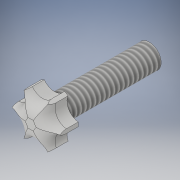
# Autodesk Inventor part: Bike Seat Bolt
Saved by Autodesk Inventor 2019 (Build 230136000, 136)
## iProperties
Created: 2020-05-31
Part Number: Bike Seat Bolt
Material: Generic
Document SubType Name: Modeling
Designer: 18186
Density: 1 g/cm^3
Appearance: Default
Author: 18186
Autodesk Inventor part; units mm, degrees
ref_plane "YZ Plane" through (0, 0, 0) normal (1, 0, 0) x (0, 1, 0)
ref_plane "XZ Plane" through (0, 0, 0) normal (0, 1, 0) x (-1, 0, 0)
ref_plane "XY Plane" through (0, 0, 0) normal (0, 0, 1) x (1, 0, 0)
sketch "Sketch1" plane through (0, 0, 0) normal (0, 0, 1) x (1, 0, 0)
  circle A0 centre (0, 0) radius 3.175
  dimension "d0" = 6.35
  constraints: 1 centre point, 1 coincident
  measures "d0" diameter of A0
extrude "Extrusion1" add sketch "Sketch1" along normal blind 25.4
sketch "Sketch2" plane through (0, 0, 25.4) normal (0, 0, 1) x (1, 0, 0)
  arc A0 (-2.7118, 5.7968) -> (2.7118, 5.7968) centre (0, 7.7132) ccw
  arc A1 (-6.3761, 0.5499) -> (-3.6643, 5.2469) centre (-6.6798, 3.8566) ccw
  arc A2 (-3.6643, -5.2469) -> (-6.3761, -0.5499) centre (-6.6798, -3.8566) ccw
  arc A3 (2.7118, -5.7968) -> (-2.7118, -5.7968) centre (0, -7.7132) ccw
  arc A4 (6.3761, -0.5499) -> (3.6643, -5.2469) centre (6.6798, -3.8566) ccw
  arc A5 (3.6643, 5.2469) -> (6.3761, 0.5499) centre (6.6798, 3.8566) ccw
  arc A6 (-2.7118, 5.7968) -> (-3.6643, 5.2469) centre (0, 0) ccw
  arc A7 (3.6643, 5.2469) -> (2.7118, 5.7968) centre (0, 0) ccw
  arc A8 (6.3761, -0.5499) -> (6.3761, 0.5499) centre (0, 0) ccw
  arc A9 (2.7118, -5.7968) -> (3.6643, -5.2469) centre (0, 0) ccw
  arc A10 (-6.3761, 0.5499) -> (-6.3761, -0.5499) centre (0, 0) ccw
  arc A11 (-3.6643, -5.2469) -> (-2.7118, -5.7968) centre (0, 0) ccw
  point P0 (-6.3761, -0.5499)
  point P1 (-2.7118, -5.7968)
  point P2 (3.6643, -5.2469)
  point P3 (6.3761, 0.5499)
  point P4 (2.7118, 5.7968)
  dimension "d7" = 360
  constraints: 24 point on circle, 12 centre point, 2 coincident, 25 other
extrude "Extrusion2" add sketch "Sketch2" along normal blind 6.35
fillet "Fillet1" radius 3.175 6 edges at (0, 4.3926, 31.75) (-3.8041, 2.1963, 31.75) (-3.8041, -2.1963, 31.75) (0, -4.3926, 31.75) (3.8041, -2.1963, 31.75) (3.8041, 2.1963, 31.75)
thread "Thread1" size "1/4-20 UNC" class "2A" standard "ANSI Unified Screw Threads" full length
body "Solid1"
